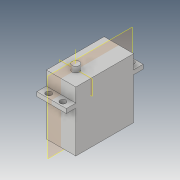
# Autodesk Inventor part: servo
Saved by Autodesk Inventor 2018 (Build 220112000, 112)
## iProperties
Created: 2020-01-08
Part Number: servo
Material: Generic
Document SubType Name: Modeling
Designer: anirudh
Density: 1 g/cm^3
Appearance: Default
Author: anirudh
Autodesk Inventor part; units mm, degrees
ref_plane "YZ Plane" through (0, 0, 0) normal (1, 0, 0) x (0, 1, 0)
ref_plane "XZ Plane" through (0, 0, 0) normal (0, 1, 0) x (-1, 0, 0)
ref_plane "XY Plane" through (0, 0, 0) normal (0, 0, 1) x (1, 0, 0)
sketch "Sketch1" plane through (0, 0, 0) normal (0, 1, 0) x (-1, 0, 0)
  line L0 (0, 0) -> (20.7, 0)
  line L1 (20.7, 0) -> (20.7, -40.6)
  line L2 (20.7, -40.6) -> (0, -40.6)
  line L3 (0, -40.6) -> (0, 0)
  dimension "d0" = 20.7
  dimension "d1" = 40.6
  constraints: 8 end point, 2 parallel, 1 horizontal, 1 perpendicular
  measures "d0" distance of L1.end L2.end
  measures "d1" distance of L0.end L1.end
extrude "Extrusion1" add sketch "Sketch1" along normal blind 29.2
sketch "Sketch2" plane through (0, 29.2, 0) normal (0, 1, 0) x (1, 0, 0)
  line L0 (0, 0) -> (0, -6.7)
  line L1 (0, -6.7) -> (-20.7, -6.7)
  line L2 (-20.7, 40.6) -> (-20.7, 0) projected
  line L3 (-20.7, -6.7) -> (-20.7, 40.6)
  line L4 (-20.7, 40.6) -> (-20.7, 47.3)
  line L5 (-20.7, 47.3) -> (0, 47.3)
  line L6 (0, 47.3) -> (0, -6.7)
  line L7 (-10.35, -6.7) -> (-15.35, -6.7)
  line L8 (-10.35, -6.7) -> (-5.35, -6.7)
  line L9 (-10.35, 47.3) -> (-15.35, 47.3)
  circle A0 centre (-15.35, -3.7) radius 2
  circle A1 centre (-5.35, -3.7) radius 2
  circle A2 centre (-15.35, 44.3) radius 2
  circle A3 centre (-5.35, 44.3) radius 2
  dimension "d6" = 5
  constraints: 18 end point, 5 point on line, 4 centre point, 4 perpendicular, 2 midpoint, 1 vertical
  measures "d6" distance of L7.start L7.end
extrude "Extrusion2" add sketch "Sketch2" along normal blind 3
sketch "Sketch3" plane through (0, 32.2, 0) normal (0, 1, 0) x (1, 0, 0)
  line L0 (0, 40.6) -> (0, 0) projected
  line L1 (-20.7, 40.6) -> (0, 40.6) projected
  line L2 (0, 0) -> (-20.7, 0)
  line L3 (-20.7, 0) -> (-20.7, 40.6)
  line L4 (-20.7, 40.6) -> (0, 40.6)
  line L5 (0, 40.6) -> (0, 0)
  constraints: 8 end point, 2 parallel, 1 horizontal, 1 perpendicular
extrude "Extrusion3" add sketch "Sketch3" along normal blind 9.8
sketch "Sketch4" plane through (0, 42, 0) normal (0, 1, 0) x (1, 0, 0)
  line L0 (0, 0) -> (-20.7, 0) projected
  line L1 (-20.7, 0) -> (0, 0)
  line L2 (0, 0) -> (0, 20.7)
  line L3 (0, 20.7) -> (-20.7, 20.7)
  line L4 (-20.7, 20.7) -> (-20.7, 0)
  line L5 (0, 0) -> (0, 40.6) projected
  circle A0 centre (-10.35, 10.35) radius 2.54
  dimension "d21" = 20.7
  dimension "d22" = 20.7
  dimension "d24" = 5.08
  constraints: 8 end point, 2 parallel, 1 centre point, 1 horizontal, 1 perpendicular
  measures "d21" distance of L3.end L2.end
  measures "d22" distance of L2.end L1.end
  measures "d24" diameter of A0
extrude "Extrusion4" add sketch "Sketch4" along normal blind 4 contours A0
ref_plane "Work Plane1" through (-10.35, 0, 0) normal (1, 0, 0) x (0, 0, -1)
ref_plane "Work Plane2" through (-20.7, 32.2, -10.3378) normal (0, 0, 1) x (1, 0, 0)
body "Solid1"
